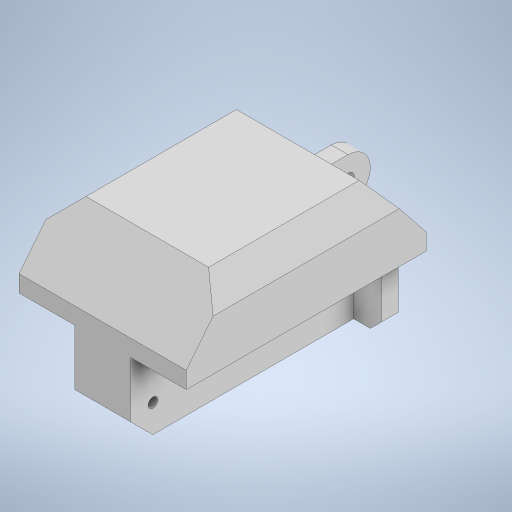
# Autodesk Inventor part: ES117_Head
Saved by Autodesk Inventor 2024 (Build 280153000, 153)
## iProperties
Created: 2023-06-04
Part Number: ES117_Head
Material: Generic
Document SubType Name: Modeling
Designer: vilas
Density: 1 g/cm^3
Appearance: Default
Author: vilas
Autodesk Inventor part; units mm, degrees
ref_plane "YZ Plane" through (0, 0, 0) normal (1, 0, 0) x (0, 1, 0)
ref_plane "XZ Plane" through (0, 0, 0) normal (0, 1, 0) x (-1, 0, 0)
ref_plane "XY Plane" through (0, 0, 0) normal (0, 0, 1) x (1, 0, 0)
sketch "Sketch1" plane through (0, 0, 0) normal (0, 0, 1) x (1, 0, 0)
  line L0 (0, 0) -> (50, 0)
  line L1 (50, 0) -> (50, 42.5)
  line L2 (50, 42.5) -> (0, 42.5)
  line L3 (0, 42.5) -> (0, 0)
  dimension "d0" = 50
  dimension "d1" = 42.5
  constraints: 8 end point, 2 parallel, 1 horizontal, 1 perpendicular
  measures "d0" distance of L2.end L1.end
  measures "d1" distance of L1.end L0.end
extrude "Extrusion1" add sketch "Sketch1" along normal blind 7.5
sketch "Sketch2" plane through (0, 0, 0) normal (0, 0, -1) x (-1, 0, 0)
  line L0 (0, 42.5) -> (0, 0) projected
  line L1 (0, 35) -> (-7.5, 35)
  line L2 (-7.5, 35) -> (-7.5, 15)
  line L3 (-7.5, 15) -> (0, 15)
  line L4 (0, 15) -> (0, 35)
  line L5 (-50, 42.5) -> (0, 42.5) projected
  line L6 (0, 0) -> (-50, 0) projected
  point P0 (0, 15)
  dimension "d4" = 7.5
  dimension "d5" = 20
  dimension "d55" = 15
  constraints: 8 end point, 2 parallel, 1 horizontal, 1 perpendicular, 1 point on line
  measures "d4" distance of L3.end L2.end
  measures "d5" distance of L2.end L1.end
  measures "d55" distance between parallel lines of L6 L3
extrude "Extrusion2" add sketch "Sketch2" along normal blind 30
fillet "Fillet1" radius 10 2 edges at (3.75, 35, -30) (3.75, 15, -30)
sketch "Sketch3" plane through (7.5, 15, 0) normal (1, 0, 0) x (0, 0, -1)
  arc A0 (20, 0) -> (20, 20) centre (20, 10) ccw projected
  line L0 (30, 10) -> (20, 10) construction
  point P0 (0, -15)
  constraints: 2 end point, 1 horizontal, 1 point on circle
hole "Hole1" at (7.5, 25, -20) direction (-1, 0, 0) diameter 4.8 end through all counterbore diameter 5.8 counterbore depth 4
chamfer "Chamfer1" distance 3 angle 45 2 edges at (3.75, 35, 0) (3.75, 15, 0)
sketch "Sketch6" plane through (0, 0, 7.5) normal (0, 0, 1) x (1, 0, 0)
  line L0 (50, 42.5) -> (0, 42.5) projected
  line L1 (25, 42.5) -> (25, -7.5) construction
  line L2 (12.5, 0) -> (12.5, 42.5)
  line L3 (12.5, 42.5) -> (37.5, 42.5)
  line L4 (37.5, 42.5) -> (37.5, 0)
  line L5 (37.5, 0) -> (12.5, 0)
  point P0 (0, 0)
  point P1 (45, 50)
  point P2 (5, 50)
  point P3 (0, 42.5)
  dimension "d43" = 50
  dimension "d44" = 42.5
  dimension "d45" = 25
  dimension "d46" = 42.5
  dimension "d47" = 12.5
  constraints: 10 end point, 2 perpendicular, 2 vertical, 2 other
  measures "d43" distance of L1.start L1.end
  measures "d44" distance of L2.start L2.end
  measures "d45" distance of L2.end L3.end
  measures "d46" distance of L3.end L4.end
  measures "d47" distance between parallel lines of L1 L2
extrude "Extrusion5" add sketch "Sketch6" along normal blind 100
sketch "Sketch10" plane through (12.5, 0, 7.5) normal (-1, 0, 0) x (0, 0, 1)
  line L0 (100, 42.5) -> (100, 0) projected
  line L1 (100, 35) -> (-7.5, 35)
  line L2 (-7.5, 35) -> (-7.5, 67.5)
  line L3 (-7.5, 67.5) -> (100, 67.5)
  line L4 (100, 67.5) -> (100, 35)
  line L5 (0, 42.5) -> (100, 42.5) projected
  point P0 (-7.5, 0)
  dimension "d66" = 107.5
  dimension "d67" = 32.5
  dimension "d68" = 7.5
  constraints: 6 end point, 2 horizontal, 1 parallel, 1 point on line, 1 vertical, 3 other
  measures "d66" distance of L3.start L3.end
  measures "d67" distance of L1.end L3.start
  measures "d68" distance between parallel lines of L1 L5
extrude "Extrusion9" add sketch "Sketch10" along normal blind 25 and the other way blind 50
chamfer "Chamfer3" distance 25 distance2 20 1 edges at (25, 67.5, 0) measured on face at (19.1667, 57.6667, 0)
chamfer "Chamfer4" distance 25 distance2 20 1 edges at (25, 67.5, 107.5) measured on face at (20.8333, 56.6667, 107.5)
chamfer "Chamfer5" distance 10 angle 45 2 edges at (-12.5, 67.5, 53.75) (62.5, 67.5, 53.75)
chamfer "Chamfer6" distance 10 angle 45 1 edges at (25, 0, 107.5)
chamfer "Chamfer7" distance 5 angle 45 2 edges at (0, 0, 3.75) (50, 0, 3.75)
sketch "Sketch11" plane through (12.5, 0, 7.5) normal (-1, 0, 0) x (0, 0, 1)
  line L0 (0, 5) -> (0, 35) projected
  line L1 (0, 12.5) -> (100, 12.5) construction
  line L2 (0, 12.5) -> (100, 12.5) construction
  line L3 (0, 0) -> (90, 0) projected
  line L4 (100, 35) -> (0, 35) projected
  line L5 (27.5, 35) -> (27.5, 0) construction
  line L6 (90, 0) -> (90, 35) construction
  line L7 (100, 35) -> (100, 10) projected
  circle A0 centre (27.5, 12.5) radius 2.15
  circle A1 centre (90, 12.5) radius 2.15
  point P0 (-7.5, 0)
  dimension "d88" = 100
  dimension "d90" = 12.5
  dimension "d91" = 27.5
  dimension "d92" = 10
  dimension "d93" = 4.3
  dimension "d94" = 4.3
  constraints: 9 point on line, 8 end point, 3 perpendicular, 2 centre point, 1 collinear, 1 horizontal
  measures "d88" distance of L1.start L1.end
  measures "d90" distance between parallel lines of L3 L1
  measures "d91" distance between parallel lines of L5 L0
  measures "d92" distance between parallel lines of L6 L7
  measures "d93" diameter of A0
  measures "d94" diameter of A1
extrude "Extrusion10" cut sketch "Sketch11" against normal through all
body "Solid1"
